Turntable Bearing_v2 (Autodesk Fusion 360 design; units mm, degrees)
Autodesk Fusion 360 part; units mm, degrees
sketch "Sketch1" plane through (0, 0, 0) normal (0, 0, 1) x (1, 0, 0)
  line L0 (-50.8, 50.8) -> (50.8, 50.8)
  line L1 (50.8, 50.8) -> (50.8, -50.8)
  line L2 (50.8, -50.8) -> (-50.8, -50.8)
  line L3 (-50.8, -50.8) -> (-50.8, 50.8)
  line L4 (-50.8, 50.8) -> (50.8, -50.8) construction
  line L5 (50.8, 50.8) -> (-50.8, -50.8) construction
  circle A0 centre (0, 0) radius 27.43
  line L6 (0, 0) -> (-40.48, 0) construction
  line L7 (-40.48, 0) -> (-40.48, -40.48) construction
  line L8 (-40.48, -40.48) -> (0, -40.48) construction
  line L9 (0, -40.48) -> (0, 0) construction
  circle A1 centre (-40.48, -40.48) radius 1.985
  circle A2 centre (-40.48, 40.48) radius 1.985
  circle A3 centre (40.48, 40.48) radius 1.985
  circle A4 centre (40.48, -40.48) radius 1.985
  circle A5 centre (0, 0) radius 45
  dimension "d1" = 101.6
  dimension "d2" = 101.6
  dimension "d3" = 54.86
  dimension "d4" = 40.48
  dimension "d5" = 40.48
  dimension "d6" = 3.97
  constraint horizontal L0
  constraint perpendicular L0 L1
  constraint parallel L0 L2
  constraint parallel L1 L3
  constraint coincident L4 A0.centre
  constraint coincident L5 A0.centre
  constraint coincident A0.centre L6.start
  constraint horizontal L6
  constraint vertical L7
  constraint horizontal L8
  constraint vertical L9
  constraint coincident L7.end L8.start
  constraint symmetric L6 A1 A2
  constraint symmetric L9 A1 A4
  constraint symmetric L9 A2 A3
  measures "d1" distance of L1.end L2.end
  measures "d2" distance of L0.end L1.end
  measures "d3" diameter of A0
  measures "d4" distance of A0.centre L6.end
  measures "d5" distance of A0.centre L8.end
  measures "d6" diameter of A1
extrude "Extrude1" add sketch "Sketch1" against normal blind 0.74 contours L0 L1 L2 L3 | A5
extrude "Extrude2" add sketch "Sketch1" along normal blind 6.65 contours A5
sketch "Sketch2" plane through (0, 0, 6.65) normal (0, 0, 1) x (-1, 0, 0)
  circle A0 centre (0, 0) radius 27.43
  circle A1 centre (0, 0) radius 45
  circle A2 centre (0, 0) radius 45
  circle A3 centre (-40.48, 40.48) radius 1.985
  circle A4 centre (40.48, 40.48) radius 1.985
  circle A5 centre (40.48, -40.48) radius 1.985
  circle A6 centre (-40.48, -40.48) radius 1.985
  line L0 (50.8, 50.8) -> (-50.8, 50.8)
  line L1 (-50.8, 50.8) -> (-50.8, -50.8)
  line L2 (-50.8, -50.8) -> (50.8, -50.8)
  line L3 (50.8, -50.8) -> (50.8, 50.8)
extrude "Extrude3" add sketch "Sketch2" along normal blind 0.74 contours A1 A2 | L0 L1 L2 L3
